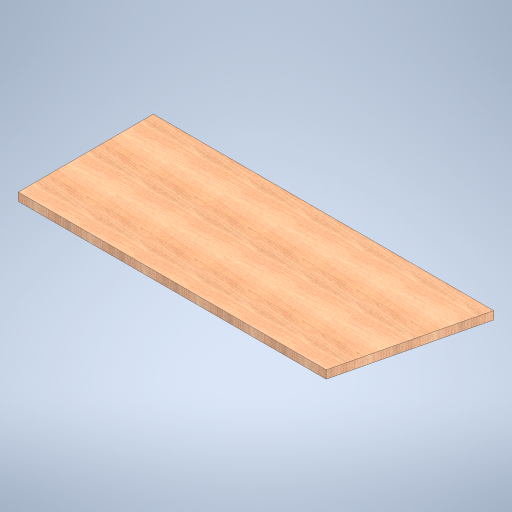
# Autodesk Inventor part: Butcher_Block--1.5_x_24_x_42.75_in
Saved by Autodesk Inventor 2024 (Build 280153000, 153)
## iProperties
Created: 2023-05-06
Part Number: Butcher_Block--1.5_x_24_x_42.75_in
Material: Wood (Birch)
Document SubType Name: Modeling
Designer: Tom
Density: 0.55 g/cm^3
Appearance: Birch - Natural Polished
Author: Tom
Autodesk Inventor part; units mm, degrees
ref_plane "YZ Plane" through (0, 0, 0) normal (1, 0, 0) x (0, 1, 0)
ref_plane "XZ Plane" through (0, 0, 0) normal (0, 1, 0) x (-1, 0, 0)
ref_plane "XY Plane" through (0, 0, 0) normal (0, 0, 1) x (1, 0, 0)
sketch "Sketch1" plane through (0, 0, 0) normal (0, 1, 0) x (-1, 0, 0)
  line L0 (0, 0) -> (-1600.2, 0)
  line L1 (-1600.2, 0) -> (-1600.2, -635)
  line L2 (-1600.2, -635) -> (0, -635)
  line L3 (0, -635) -> (0, 0)
  dimension "d6" = 635
  dimension "d10" = 1600.2
  constraints: 8 end point, 2 parallel, 1 coincident, 1 horizontal, 1 perpendicular
  measures "d6" distance of L2.end L0.start
  measures "d10" distance of L1.end L2.end
extrude "Extrusion1" add sketch "Sketch1" along normal blind 38.1
sketch "Sketch2" plane through (0, 38.1, 0) normal (0, 1, 0) x (1, 0, 0)
  line L0 (1600.2, 0) -> (1600.2, 635) projected
  line L1 (1600.2, 635) -> (1447.8, 0)
  line L2 (0, 0) -> (1600.2, 0) projected
  line L3 (1447.8, 0) -> (1600.2, 0)
  line L4 (1600.2, 0) -> (1600.2, 635)
  dimension "d11" = 152.4
  constraints: 6 end point, 1 collinear, 1 perpendicular, 1 point on line
  measures "d11" distance of L1.end L0.start
extrude "Extrusion2" cut sketch "Sketch2" against normal through all
body "Solid1"
